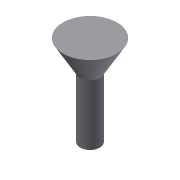
# Autodesk Inventor part: Vane_Stud
Saved by Autodesk Inventor 2022 (Build 260148000, 148)
## iProperties
Created: 2005-10-19
Part Number: Vane_Stud
Document SubType Name: Modeling
Designer: landrews
Density: 1 g/cm^3
Material: Generic
Appearance: Default
Author: landrews
Autodesk Inventor part; units mm, degrees
ref_plane "YZ Plane" through (0, 0, 0) normal (1, 0, 0) x (0, 1, 0)
ref_plane "XZ Plane" through (0, 0, 0) normal (0, 1, 0) x (-1, 0, 0)
ref_plane "XY Plane" through (0, 0, 0) normal (0, 0, 1) x (1, 0, 0)
sketch "Sketch1" plane through (0, 0, 0) normal (1, 0, 0) x (0, 1, 0)
  line L0 (0, 1.2573) -> (0, -4.6101) projected
  line L1 (-15.367, 0) -> (4.191, 0) projected
  line L2 (0, 0) -> (0, -4.191)
  line L3 (0, -4.191) -> (-4.6194, -1.524)
  line L4 (-4.6194, -1.524) -> (-13.97, -1.524)
  line L5 (-13.97, -1.524) -> (-13.97, 0)
  line L6 (-13.97, 0) -> (0, 0)
  dimension "d0" = 8.382
  dimension "d1" = 60
  dimension "d2" = 13.97
  dimension "d3" = 3.048
  constraints: 10 end point, 4 point on line, 2 perpendicular, 1 collinear
  measures "d0" diameter of L2.end L1
  measures "d1" angle of L3 L0
  measures "d2" distance between parallel lines of L5 L0
  measures "d3" diameter of L4 L6
revolve "Revolution1" add sketch "Sketch1" angle 360 about axis through (0, 0, 0) along (0, 1, 0)
body "Solid1"
